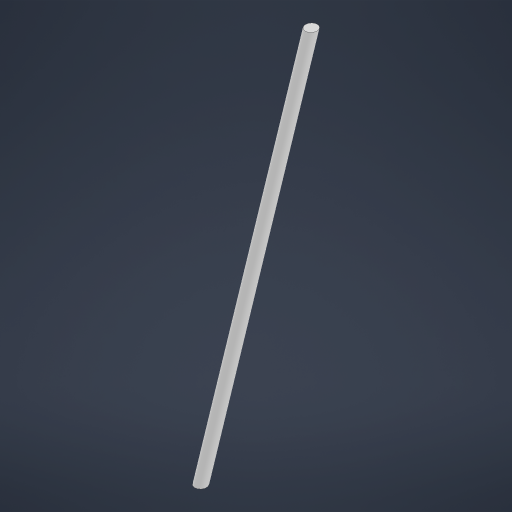
# Autodesk Inventor part: Leg_Mockup
Saved by Autodesk Inventor 2023 (Build 270158000, 158)
## iProperties
Created: 2023-06-08
Part Number: Leg_Mockup
Material: Generic
Document SubType Name: Modeling
Designer: dzw04
Density: 1 g/cm^3
Appearance: Default
Author: dzw04
Autodesk Inventor part; units mm, degrees
ref_plane "YZ Plane" through (0, 0, 0) normal (1, 0, 0) x (0, 1, 0)
ref_plane "XZ Plane" through (0, 0, 0) normal (0, 1, 0) x (-1, 0, 0)
ref_plane "XY Plane" through (0, 0, 0) normal (0, 0, 1) x (1, 0, 0)
sketch "Sketch1" plane through (0, 0, 0) normal (1, 0, 0) x (0, 1, 0)
  line L0 (0, 0) -> (-475.5283, 154.5085)
  line L1 (0, 0) -> (500, 0) construction
  line L2 (-470.584, 169.7254) -> (2.5342, 16)
  line L3 (2.5342, 16) -> (500, 16)
  line L4 (0, 0) -> (0, 16.8234)
  line L5 (-470.584, 169.7254) -> (-470.584, 152.902)
  dimension "d0" = 500
  dimension "d1" = 162
  dimension "d2" = 16
  constraints: 12 end point, 2 point on line, 1 equal length, 1 horizontal, 1 parallel, 1 vertical, 1 other
  measures "d0" distance of L0.start L0.end
  measures "d1" angle of L1 L0
  measures "d2" distance between parallel lines of L0 L2
extrude "Extrusion1" add sketch "Sketch1" along normal blind 16
fillet "Fillet1" radius 8 4 edges at (16, -235.292, 76.451) (0, -235.292, 76.451) (16, -235.292, 93.2744) (0, -235.292, 93.2744)
body "Solid1"
